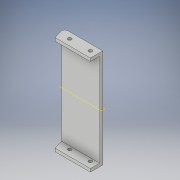
# Autodesk Inventor part: cameraMount
Saved by Autodesk Inventor 2018 (Build 220112000, 112)
## iProperties
Created: 2020-01-14
Part Number: cameraMount
Material: Generic
Document SubType Name: Modeling
Designer: anirudh.bali
Density: 1 g/cm^3
Appearance: Default
Author: anirudh.bali
Autodesk Inventor part; units mm, degrees
ref_plane "YZ Plane" through (0, 0, 0) normal (1, 0, 0) x (0, 1, 0)
ref_plane "XZ Plane" through (0, 0, 0) normal (0, 1, 0) x (-1, 0, 0)
ref_plane "XY Plane" through (0, 0, 0) normal (0, 0, 1) x (1, 0, 0)
sketch "Sketch1" plane through (0, 0, 0) normal (0, 1, 0) x (-1, 0, 0)
  circle A0 centre (0, 0) radius 1.75
  line L0 (-27.6489, -6.35) -> (8.2567, -6.35)
  line L1 (0, 6.35) -> (8.675, 6.35)
  circle A1 centre (-21.2989, 0) radius 1.75
  line L2 (-27.6489, 0) -> (-27.6489, 6.35)
  line L3 (-27.6489, 6.35) -> (0.5716, 6.35)
  line L4 (-27.6489, 0) -> (-27.6489, -6.35)
  arc A2 (8.2567, -6.35) -> (11.314, -2.3183) centre (8.2567, -3.175) ccw
  line L5 (-27.6489, -6.35) -> (8.2567, -6.35)
  arc A3 (8.2567, -6.35) -> (11.314, -2.3183) centre (8.2567, -3.175) ccw
  arc A4 (11.314, -2.3183) -> (8.675, 6.35) centre (-184.3483, -57.15) ccw
  constraints: 12 end point, 6 point on circle, 5 centre point, 3 point on line, 1 coincident, 1 perpendicular, 1 tangent
extrude "Extrusion1" add sketch "Sketch1" along normal blind 3.175
sketch "Sketch2" plane through (0, 3.175, 0) normal (0, 1, 0) x (1, 0, 0)
  line L0 (27.6489, 6.35) -> (-8.2567, 6.35) projected
  arc A0 (-8.2567, 6.35) -> (-11.314, 2.3183) centre (-8.2567, 3.175) ccw projected
  line L1 (27.6489, 6.35) -> (-8.2567, 6.35)
  line L2 (-11.4317, 3.175) -> (27.6489, 3.175)
  line L3 (27.6489, 3.175) -> (27.6489, 6.35)
  arc A1 (-8.2567, 6.35) -> (-11.4317, 3.175) centre (-8.2567, 3.175) ccw
  point P0 (0, 0)
  constraints: 7 end point, 3 point on circle, 1 centre point, 1 coincident, 1 horizontal, 1 parallel
extrude "Extrusion2" add sketch "Sketch2" along normal blind 47.625
ref_plane "Work Plane1" through (0, 50.8, 0) normal (0, 1, 0) x (1, 0, 0)
mirror "Mirror1" about plane through (0, 50.8, 0) normal (0, 1, 0) of "Extrusion1", "Extrusion2"
sketch "Sketch4" plane through (0, 50.8, 0) normal (0, 1, 0) x (1, 0, 0)
  line L0 (27.6489, 6.35) -> (-8.2567, 6.35) projected
  arc A0 (-19.3411, 37.8477) -> (27.6489, 6.35) centre (27.6489, 57.15) ccw
  line L1 (27.6489, 6.35) -> (-8.2567, 6.35)
  arc A1 (-19.3411, 16.3849) -> (-8.2567, 6.35) centre (27.6489, 57.15) ccw
  line L2 (-19.3411, 16.3849) -> (-19.3411, 37.8477)
  point P0 (0, 0)
  constraints: 5 point on circle, 4 end point, 2 centre point, 1 coincident, 1 vertical
extrude "Extrusion3" add sketch "Sketch4" along normal mid plane 25.4
body "Solid1"
